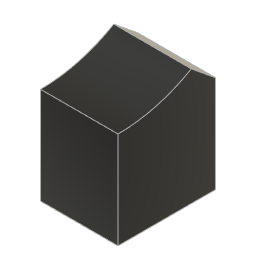
Q1 Table Lamp (Autodesk Fusion 360 archive; units mm, degrees)
design "Switch"
Autodesk Fusion 360 part; units mm, degrees
sketch "Sketch1" plane through (0, 0, 0) normal (1, 0, 0) x (0, 1, 0)
  line L0 (0, 0) -> (0, 10)
  arc A0 (0, 10) -> (7.564, 12.0468) centre (0, 25) ccw
  line L1 (10.0627, 0) -> (10.0627, 10)
  line L2 (7.564, 12.0468) -> (10.0627, 10)
  line L3 (0, 0) -> (10.0627, 0)
  dimension "d1" = 10
  dimension "d3" = 15
  dimension "d7" = 3.23
  dimension "d8" = 10
  constraint coincident L0.start L3.start
  constraint vertical L0
  constraint vertical L0.end A0.centre
  constraint vertical L1
  constraint horizontal L0.start L1.start
  measures "d1" distance of L0.start L0.end
  measures "d3" radius of A0
  measures "d7" distance of A0.end L1.end
  measures "d8" distance of L1.start L1.end
extrude "Extrude1" add sketch "Sketch1" along normal blind 8

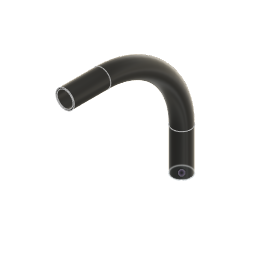
design "Pipe"
Autodesk Fusion 360 part; units mm, degrees
sketch "Sketch1" plane through (0, 0, 0) normal (1, 0, 0) x (0, 1, 0)
  line L0 (0, 0) -> (0, 68.58)
  line L1 (-130.42, 199) -> (-190, 199)
  arc A0 (0, 68.58) -> (-130.42, 199) centre (-130.42, 68.58) ccw
  point P0 (0, 68.58)
  point P1 (-140, 199)
  dimension "d1" = 68.58
  dimension "d2" = 50
  dimension "d4" = 130.42
  constraint coincident L0.start origin
  constraint vertical L0
  constraint horizontal L1
  constraint coincident P1 L1
  constraint coincident P0 L0
  constraint tangent L1 A0
  constraint tangent L0 A0
  constraint coincident P0 L0.end
  measures "d1" distance of L0.start P0
  measures "d2" distance of P1 L1.end
  measures "d4" radius of A0
sketch "Sketch2" plane through (0, 0, 0) normal (0, 0, 1) x (1, 0, 0)
  circle A0 centre (0, 0) radius 15
  dimension "d5" = 30
  constraint coincident A0.centre origin
  measures "d5" diameter of A0
ref_plane "WorkPlane1" through (0, -190, 199) normal (0, -1, 0) x (1, 0, 0)
sketch "Sketch3" plane through (0, -190, 199) normal (0, -1, 0) x (1, 0, 0)
  circle A0 centre (0, 0) radius 15
  dimension "d7" = 30
  constraint coincident A0.centre origin
  measures "d7" diameter of A0
sweep "Sweep1" add profiles "Sketch3" path "Sketch1" along L0 A0 L1 section 1
shell "Shell1" thickness 2 removed faces 1 at (-5.6583, -190, 198.4751)
